# Autodesk Inventor part: Roller Chain Sprocket2
Saved by Autodesk Inventor 2016 (Build 200138000, 138)
## iProperties
Created: 2016-05-21
Part Number: Roller Chain Sprocket2
Material: Steel
Document SubType Name: Modeling
Designer: Henrik Samuelsson
Density: 1 g/cm^3
Appearance: Steel
CustomPartVersion: 1
Author: Henrik Samuelsson
Autodesk Inventor part; units mm, degrees
ref_plane "YZ Plane" through (0, 0, 0) normal (1, 0, 0) x (0, 1, 0)
ref_plane "XZ Plane" through (0, 0, 0) normal (0, 1, 0) x (-1, 0, 0)
sketch "Theoretical Tooth Profile" plane through (0, 0, 0) normal (0, 0, 1) x (1, 0, 0)
  circle A0 centre (0, 0) radius 86.453 construction
  line L0 (0, 0) -> (0, 86.453) construction
  line L1 (0, 0) -> (9.5105, 85.9283) construction
  circle A1 centre (0, 0) radius 89.1792
  arc A2 (-2.5926, 84.5657) -> (2.5926, 84.5657) centre (0, 86.453) ccw
  line L2 (0, 86.453) -> (9.5105, 85.9283) construction
  line L3 (0, 86.453) -> (4.1071, 89.4427) construction
  line L4 (4.1071, 89.4427) -> (-3.7266, 86.74) construction
  arc A3 (4.7899, 89.0505) -> (4.0349, 87.6336) centre (8.8765, 85.9632) ccw
  arc A4 (-4.0349, 87.6336) -> (-4.7899, 89.0505) centre (-8.8765, 85.9632) ccw
  line L5 (-8.8765, 85.9632) -> (-4.0349, 87.6336) construction
  arc A5 (-3.7266, 86.74) -> (-2.5926, 84.5657) centre (4.1071, 89.4427) ccw
  line L6 (-3.7266, 86.74) -> (-4.0349, 87.6336)
  arc A6 (2.5926, 84.5657) -> (3.7266, 86.74) centre (-4.1071, 89.4427) ccw
  line L7 (4.0349, 87.6336) -> (3.7266, 86.74)
  line L8 (0, 0) -> (4.9127, 89.0438) construction
  point P0 (4.7553, 86.1906)
  dimension "d0" = 172.9059
  dimension "d2" = 6.316
  dimension "d3" = 3.2067
  dimension "d10" = 126.053
  dimension "d11" = 17.017
  dimension "d12" = 5.08
  dimension "d13" = 8.2867
  dimension "d14" = 8.89
  dimension "d23" = 2.8575
  constraints: 18 end point, 15 point on circle, 7 centre point, 3 coincident, 3 point on line, 3 symmetric about line, 3 tangent, 1 equal radius, 1 midpoint, 1 parallel, 1 vertical, 1 other
  measures "d0" diameter of A0
  measures "d2" angle of L1 L0
  measures "d3" radius of A2
  measures "d10" angle of L3 L0
  measures "d11" angle of L4 L3
  measures "d12" distance of L2.start L3.end
  measures "d13" distance of L3.end L4.end
  measures "d14" distance of A3.centre L0.end
  measures "d23" distance from line of L8.end L2
sketch "Tooth Profile" plane through (0, 0, 0) normal (0, 0, 1) x (1, 0, 0)
  arc A0 (-2.998, 85.3148) -> (2.998, 85.3148) centre (0, 86.453) ccw
  arc A1 (4.6177, 89.0596) -> (2.998, 85.3148) centre (45.0288, 69.3576) ccw
  arc A2 (-2.998, 85.3148) -> (-4.6177, 89.0596) centre (-45.0288, 69.3576) ccw
  line L0 (0, 0) -> (0, 86.453) construction
  line L1 (0, 86.453) -> (2.998, 85.3148) construction
  line L2 (0, 86.453) -> (-2.998, 85.3148) construction
  circle A3 centre (0, 0) radius 89.1792 projected
  dimension "d44" = 138.421
  dimension "d45" = 44.958
  dimension "d46" = 3.2067
  constraints: 9 point on circle, 6 end point, 3 centre point, 2 tangent, 1 coincident, 1 equal radius, 1 vertical, 1 other
  measures "d44" angle of L2 L1
  measures "d45" radius of A1
  measures "d46" radius of A0
sketch "Section Profile" plane through (0, 0, 0) normal (1, 0, 0) x (0, 1, 0)
  line L0 (89.1792, 0) -> (-89.1792, 0) projected
  line L1 (77.8455, 2.6598) -> (-77.8455, 2.6598)
  line L2 (-77.8455, 2.6598) -> (-77.8455, -2.6598)
  line L3 (-77.8455, -2.6598) -> (77.8455, -2.6598)
  line L4 (77.8455, -2.6598) -> (77.8455, 2.6598)
  line L5 (77.8455, 2.6598) -> (89.1792, 2.6598) construction
  line L6 (89.1792, 2.6598) -> (89.1792, -2.6598) construction
  line L7 (89.1792, -2.6598) -> (77.8455, -2.6598) construction
  line L8 (77.8455, -2.6598) -> (77.8455, 2.6598)
  arc A0 (89.1792, 1.4692) -> (84.5679, 2.6598) centre (84.5679, -6.8652) ccw
  arc A1 (84.5679, -2.6598) -> (89.1792, -1.4692) centre (84.5679, 6.8652) ccw
  line L9 (84.5679, 2.6598) -> (0, 2.6598)
  line L10 (0, 2.6598) -> (0, -2.6598)
  line L11 (0, -2.6598) -> (84.5679, -2.6598)
  line L12 (0, 2.6598) -> (0, -2.6598)
  line L13 (89.1792, 1.4692) -> (89.1792, -1.4692)
  point P0 (0, 0)
  point P1 (0, 0)
  dimension "d30" = 5.3196
  dimension "d31" = 155.691
  dimension "d32" = 5.3196
  dimension "d33" = 1.1906
  dimension "d34" = 9.525
  dimension "d43" = 2.6598
  constraints: 26 end point, 7 midpoint, 5 perpendicular, 4 parallel, 4 point on circle, 3 point on line, 3 symmetric about line, 2 centre point, 2 horizontal, 2 tangent, 1 collinear, 1 other
  measures "d30" distance between parallel lines of L7 L5
  measures "d31" distance between parallel lines of L2 L4
  measures "d32" distance between parallel lines of L3 L1
  measures "d33" distance from line of L13.start L5
  measures "d34" radius of A0
  measures "d43" distance between parallel lines of L3 L0
revolve "Shroud" add sketch "Section Profile" angle 360 about axis through (0, 0, 2.6598) along (0, 0, -1) contours L10 L3 L2 L0 | L0 L2 L1 L10
revolve "Strand" add sketch "Section Profile" angle 360 about axis through (0, 0, 2.6598) along (0, 0, -1) contours L13 A1 L11 L4 L0 | L0 L4 L9 A0 L13 | L4 L3 L10 L0 | L0 L10 L1 L4
pattern_of_one "Strand Pattern"
extrude "Theoretical Tooth" cut sketch "Theoretical Tooth Profile" along normal through all both and the other way through all contours A3 L7 A6 A2 A5 L6 A4 A1 picked at (0, 87.192)
extrude "Tooth" [suppressed]
pattern_circular "Tooth Pattern" count 57 over 360 about axis through (0, 0, -10) along (0, 0, 1) of "Theoretical Tooth"
ref_plane "Timing Plane" through (0, 86.453, 0) normal (1, 0, 0) x (0, 1, 0)
equation "\"d3\" = 0.5 * da_Dr + da_SC"
equation "\"d12\" = 0.8 * da_Dr"
equation "\"d13\" = 1.3 * da_Dr + da_SC"
equation "\"d14\" = 1.4 * da_Dr"
equation "\"d23\" = da_Ha"
equation "\"d44\" = da_Alfa"
equation "\"d45\" = da_Re"
equation "\"d46\" = da_Ri"
equation "\"d30\" = da_Bf"
equation "\"d31\" = da_Ds"
equation "\"d32\" = da_Bs"
equation "\"d33\" = da_Ba"
equation "\"d34\" = da_Rx"
equation "\"d40\" = da_pt"
equation "\"form_type\" = 0"
equation "\"da_p\" = 9.525"
equation "\"da_Dr\" = 6.35"
equation "\"da_SC\" = 0.03175"
equation "\"da_Ha\" = 2.8575"
equation "\"da_pt\" = 10.24"
equation "\"da_Bf\" = 5.3196"
equation "\"da_Ba\" = 1.19063"
equation "\"da_Rx\" = 9.525"
equation "\"da_Ra\" = 0.381"
equation "\"da_Bs\" = 5.3196"
equation "\"da_Ds\" = 155.69097"
equation "\"da_Re\" = 44.958"
equation "\"da_Ri\" = 3.20675"
equation "\"da_Alfa\" = 138.421deg"
body "Solid1"
